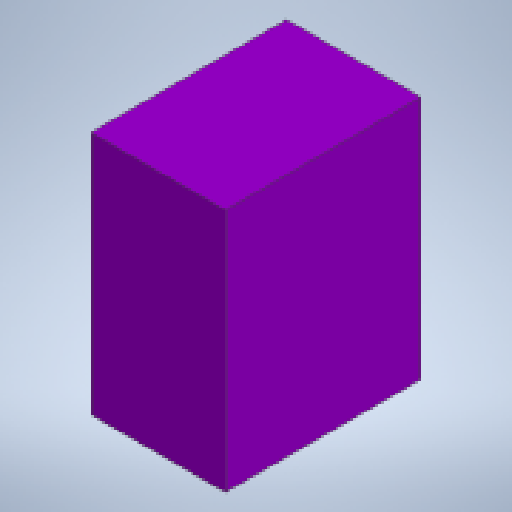
# Autodesk Inventor part: GPHN barrel
Saved by Autodesk Inventor 2025.4 (Build 294407000, 407)
## iProperties
Created: 2025-03-29
Part Number: GPHN barrel
Material: Generic
Document SubType Name: Modeling
Designer: pokla
Density: 1 g/cm^3
Appearance: Default
Author: pokla
Autodesk Inventor part; units mm, degrees
ref_plane "YZ Plane" through (0, 0, 0) normal (1, 0, 0) x (0, 1, 0)
ref_plane "XZ Plane" through (0, 0, 0) normal (0, 1, 0) x (-1, 0, 0)
ref_plane "XY Plane" through (0, 0, 0) normal (0, 0, 1) x (1, 0, 0)
sketch "Sketch1" plane through (0, 0, 0) normal (0, 0, 1) x (1, 0, 0)
  line L0 (-275, 400) -> (275, 400)
  line L1 (275, 400) -> (275, -400)
  line L2 (275, -400) -> (-275, -400)
  line L3 (-275, -400) -> (-275, 400)
  line L4 (-275, -400) -> (275, 400) construction
  point P0 (0, 0)
  point P1 (0, 0)
  dimension "d0" = 550
  dimension "d1" = 800
  constraints: 10 end point, 2 parallel, 1 coincident, 1 horizontal, 1 midpoint, 1 perpendicular
  measures "d0" distance of L0.start L0.end
  measures "d1" distance between parallel lines of L2 L0
extrude "Extrusion1" add sketch "Sketch1" along normal blind 1000
equation "\"d0\" = Длина"
equation "\"d1\" = Ширина"
equation "\"d2\" = Высота"
equation "\"Длина\" = 550"
equation "\"Ширина\" = 800"
equation "\"Высота\" = 1000"
body "Solid1"
